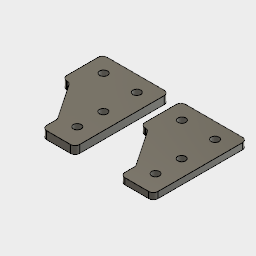
Z_Bottom_Brace_Stronger_v3 (Autodesk Fusion 360 design; units mm, degrees)
Autodesk Fusion 360 part; units mm, degrees
sketch "Sketch2" plane through (0, 0, 0) normal (0, 1, 0) x (1, 0, 0)
  line L0 (-12, 25) -> (24.3714, 25)
  line L1 (27.3714, 22) -> (27.3714, -32)
  line L2 (24.3714, -35) -> (9.1857, -35)
  line L3 (-15, 1.967) -> (-15, 22)
  circle A0 centre (16.7786, -22.9968) radius 2.5
  circle A1 centre (16.7786, -6.2991) radius 2.5
  circle A2 centre (16.7786, 15.0225) radius 2.5
  circle A3 centre (-4.4071, 15.0225) radius 2.5
  arc A4 (-12, 25) -> (-15, 22) centre (-12, 22) ccw
  arc A5 (27.3714, 22) -> (24.3714, 25) centre (24.3714, 22) ccw
  arc A6 (24.3714, -35) -> (27.3714, -32) centre (24.3714, -32) ccw
  arc A7 (6.1857, -32) -> (9.1857, -35) centre (9.1857, -32) ccw
  arc A8 (-15, 1.967) -> (-12, -1.033) centre (-12, 1.967) ccw
  line L4 (-9.1334, -2.3557) -> (5.673, -24.3128)
  line L5 (-12, -1.033) -> (-11.6207, -1.033)
  line L6 (6.1857, -32) -> (6.1857, -25.9901)
  arc A9 (-9.1334, -2.3557) -> (-11.6207, -1.033) centre (-11.6207, -4.033) ccw
  arc A10 (6.1857, -25.9901) -> (5.673, -24.3128) centre (3.1857, -25.9901) ccw
  dimension "d1" = 5
  dimension "d2" = 5
  dimension "d3" = 5
  dimension "d4" = 5
  dimension "d5" = 3
  dimension "d9" = 3
  measures "d1" diameter of A0
  measures "d2" diameter of A1
  measures "d3" diameter of A2
  measures "d4" diameter of A3
  measures "d5" radius of A4
  measures "d9" radius of A9
extrude "Extrude1" add sketch "Sketch2" along normal blind 5 makes body 1
copy_body "CopyPasteBodies1" bodies 1 makes body 2
move_body "Move1" bodies 2 to x (1, 0, 0) y (0, 1, 0) z (0, 0, 1) at (50, 0, 0)
move_face "OffsetFaces1" offset -1 1 faces at (53.6431, 5, 11.2348) on bodies 2
named bodies: "5mm", "4mm"
